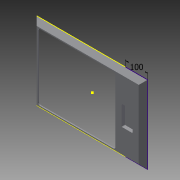
# Autodesk Inventor part: SitzFläche
Saved by Autodesk Inventor 2018.2 (Build 222227000, 227)
## iProperties
Created: 2019-02-06
Part Number: SitzFläche
Material: Generisch
Document SubType Name: Modeling
Designer: Lolob
Density: 1 g/cm^3
Appearance: Vorgabe
Author: Lolob
Autodesk Inventor part; units mm, degrees
ref_plane "YZ Plane" through (0, 0, 0) normal (1, 0, 0) x (0, 1, 0)
ref_plane "XZ Plane" through (0, 0, 0) normal (0, 1, 0) x (-1, 0, 0)
ref_plane "XY Plane" through (0, 0, 0) normal (0, 0, 1) x (1, 0, 0)
sketch "Skizze1" plane through (0, 0, 0) normal (0, 1, 0) x (-1, 0, 0)
  line L0 (350, 0) -> (-350, 0) projected
  line L1 (0, -245) -> (0, 245) projected
  line L2 (250, 175) -> (-250, 175)
  line L3 (-250, 175) -> (-250, -175)
  line L4 (-250, -175) -> (250, -175)
  line L5 (250, -175) -> (250, 175)
  point P0 (0, 0)
  dimension "d0" = 350
  dimension "d1" = 500
  constraints: 8 end point, 2 parallel, 1 horizontal, 1 perpendicular, 2 other
  measures "d0" distance of L2.end L3.end
  measures "d1" distance of L2.start L2.end
extrude "Extrusion1" add sketch "Skizze1" along normal blind 20
chamfer "Fase1" distance 20 angle 45 4 edges at (-250, 0, 0) (0, 0, 175) (250, 0, 0) (0, 0, -175)
sketch "Skizze2" plane through (0, 20, 0) normal (0, 1, 0) x (1, 0, 0)
  line L0 (250, -175) -> (250, 175) projected
  line L1 (250, 175) -> (-250, 175) projected
  line L2 (-250, -175) -> (250, -175) projected
  line L3 (250, 175) -> (150, 175)
  line L4 (150, 175) -> (150, -175)
  line L5 (150, -175) -> (250, -175)
  line L6 (250, -175) -> (250, 175)
  point P0 (0, 0)
  dimension "d7" = 100
  constraints: 8 end point, 2 parallel, 1 horizontal, 1 perpendicular, 1 point on line
  measures "d7" distance of L5.end L4.end
sketch "Skizze3" plane through (0, 20, 0) normal (0, 1, 0) x (1, 0, 0)
  line L0 (-250, 175) -> (-250, -175) projected
  line L1 (150, 175) -> (150, -175) projected
  line L2 (-230, 155) -> (-230, -155) projected
  line L3 (-230, -155) -> (230, -155) projected
  line L4 (-220, 155) -> (120, 155)
  line L5 (130, 145) -> (130, -145)
  line L6 (120, -155) -> (-220, -155)
  line L7 (-230, -145) -> (-230, 145)
  arc A0 (-220, 155) -> (-230, 145) centre (-220, 145) ccw
  arc A1 (130, 145) -> (120, 155) centre (120, 145) ccw
  arc A2 (120, -155) -> (130, -145) centre (120, -145) ccw
  arc A3 (-230, -145) -> (-220, -155) centre (-220, -145) ccw
  point P0 (0, 0)
  point P1 (130, -155)
  point P2 (130, 155)
  dimension "d8" = 20
  dimension "d29" = 10
  dimension "d30" = 10
  constraints: 8 end point, 8 point on circle, 8 tangent, 7 point on line, 4 centre point, 2 equal radius, 2 parallel, 1 horizontal, 1 perpendicular
  measures "d8" distance between parallel lines of L1 L5
  measures "d29" radius of A0
  measures "d30" radius of A1
extrude "Extrusion2" cut sketch "Skizze3" against normal blind 15 contours A0 L4 A1 L5 A2 L3 A3 L2
sketch "Skizze4" plane through (0, 5, 0) normal (0, 1, 0) x (1, 0, 0)
  line L0 (130, 145) -> (130, -145) projected
  line L1 (-220, 155) -> (120, 155) projected
  line L2 (-215, 150) -> (115, 150)
  line L3 (125, 140) -> (125, -140)
  line L4 (115, -150) -> (-215, -150)
  line L5 (-225, -140) -> (-225, 140)
  arc A0 (-220, 155) -> (-230, 145) centre (-220, 145) ccw projected
  line L6 (-230, -145) -> (-230, 145) projected
  arc A1 (-230, -145) -> (-220, -155) centre (-220, -145) ccw projected
  line L7 (120, -155) -> (-220, -155) projected
  arc A2 (120, -155) -> (130, -145) centre (120, -145) ccw projected
  arc A3 (130, 145) -> (120, 155) centre (120, 145) ccw projected
  arc A4 (-215, 150) -> (-225, 140) centre (-215, 140) ccw
  arc A5 (125, 140) -> (115, 150) centre (115, 140) ccw
  arc A6 (115, -150) -> (125, -140) centre (115, -140) ccw
  arc A7 (-225, -140) -> (-215, -150) centre (-215, -140) ccw
  point P0 (0, 0)
  point P1 (-225, 150)
  point P2 (125, -150)
  point P3 (125, 150)
  point P4 (-225, -150)
  dimension "d11" = 5
  dimension "d13" = 5
  dimension "d31" = 10
  constraints: 8 end point, 8 point on circle, 8 point on line, 8 tangent, 4 centre point, 3 equal radius, 2 parallel, 1 horizontal, 1 perpendicular
  measures "d11" distance between parallel lines of L1 L2
  measures "d13" distance between parallel lines of L0 L3
  measures "d31" radius of A4
extrude "Extrusion3" cut sketch "Skizze4" against normal blind 5 contours L2 A5 L3 A6 L4 A7 L5 A4
sketch "Skizze5" plane through (0, 20, 0) normal (0, 1, 0) x (1, 0, 0)
  line L0 (-230, 165) -> (130, 165)
  line L1 (140, 155) -> (140, -155)
  line L2 (130, -165) -> (-230, -165)
  line L3 (-240, -155) -> (-240, 155)
  line L4 (-250, 175) -> (-250, -175) projected
  line L5 (250, 175) -> (-250, 175) projected
  line L6 (125, 140) -> (125, -140) projected
  line L7 (-250, -175) -> (250, -175) projected
  arc A0 (-230, 165) -> (-240, 155) centre (-230, 155) ccw
  arc A1 (140, 155) -> (130, 165) centre (130, 155) ccw
  arc A2 (130, -165) -> (140, -155) centre (130, -155) ccw
  arc A3 (-240, -155) -> (-230, -165) centre (-230, -155) ccw
  point P0 (0, 0)
  point P1 (-240, 165)
  point P2 (140, -165)
  point P3 (140, 165)
  point P4 (-240, -165)
  point P5 (125, 150)
  point P6 (125, -150)
  dimension "d17" = 10
  dimension "d18" = 10
  dimension "d19" = 15
  dimension "d20" = 10
  dimension "d32" = 10
  constraints: 8 end point, 8 point on circle, 8 point on line, 8 tangent, 4 centre point, 3 equal radius, 2 parallel, 1 horizontal, 1 perpendicular
  measures "d17" distance between parallel lines of L4 L3
  measures "d18" distance between parallel lines of L5 L0
  measures "d19" distance between parallel lines of L6 L1
  measures "d20" distance between parallel lines of L7 L2
  measures "d32" radius of A0
extrude "Extrusion4" cut sketch "Skizze5" against normal blind 10
sketch "Skizze6" plane through (0, 0, 0) normal (0, -1, 0) x (1, 0, 0)
  line L0 (125, 140) -> (125, -140) projected
  line L1 (230, 155) -> (230, -155) projected
  line L2 (-350, 0) -> (350, 0) projected
  line L3 (152.5, 42.534) -> (202.5, 42.534)
  line L4 (202.5, 42.534) -> (202.5, -47.466)
  line L5 (202.5, -47.466) -> (152.5, -47.466)
  line L6 (152.5, -47.466) -> (152.5, 42.534)
  point P0 (0, 0)
  point P1 (125, 150)
  point P2 (125, -150)
  dimension "d23" = 50
  dimension "d24" = 90
  dimension "d25" = 27.5
  constraints: 8 end point, 2 parallel, 1 horizontal, 1 perpendicular
  measures "d23" distance of L3.start L3.end
  measures "d24" distance of L3.end L4.end
  measures "d25" distance between parallel lines of L1 L4
extrude "Extrusion5" cut sketch "Skizze6" against normal blind 15
fillet "Rundung1" radius 4 4 edges at (152.5, 7.5, 42.534) (202.5, 7.5, 42.534) (202.5, 7.5, -47.466) (152.5, 7.5, -47.466)
